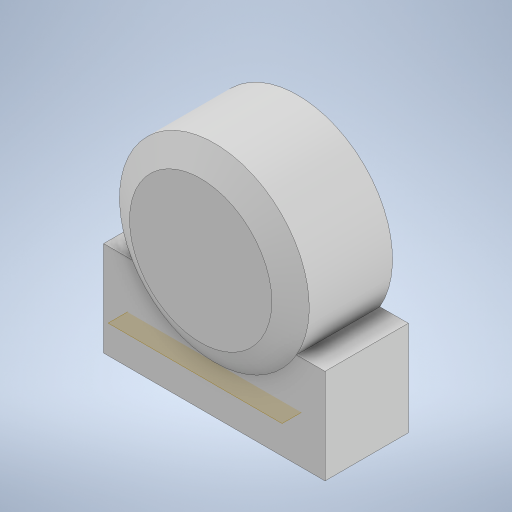
# Autodesk Inventor part: transmission_box_l_to_r
Saved by Autodesk Inventor 2023 (Build 270158000, 158)
## iProperties
Created: 2023-12-09
Part Number: transmission_box_l_to_r
Material: Generic
Document SubType Name: Modeling
Designer: Peter
Density: 1 g/cm^3
Appearance: Default
Author: Peter
Autodesk Inventor part; units mm, degrees
ref_plane "YZ Plane" through (0, 0, 0) normal (1, 0, 0) x (0, 1, 0)
ref_plane "XY Plane" through (0, 0, 0) normal (0, 0, 1) x (1, 0, 0)
sketch "Sketch2" plane through (0, 0, 0) normal (0, 0, 1) x (1, 0, 0)
  circle A0 centre (0, 0) radius 76.2
  dimension "d7" = 152.4
  constraints: 1 centre point, 1 coincident
  measures "d7" diameter of A0
extrude "Extrusion2" add sketch "Sketch2" along normal blind 88.9
chamfer "Chamfer1" distance 19.05 angle 30 1 edges at (-76.2, 0, 88.9) measured on face at (-0.8389, -20.4706, 88.9)
chamfer "Chamfer2" distance 19.05 angle 30 1 edges at (-76.2, 0, 0) measured on face at (-0.8389, -20.4706, 0)
ref_plane "Work Plane1" through (0, -76.2, 0) normal (0, 1, 0) x (-1, 0, 0)
sketch "Sketch10" plane through (0, -76.2, 0) normal (0, 1, 0) x (-1, 0, 0)
  line L0 (88.9, 77.9015) -> (-88.9, 77.9015)
  line L1 (-88.9, 77.9015) -> (-88.9, 10.9985)
  line L2 (-88.9, 10.9985) -> (88.9, 10.9985)
  line L3 (88.9, 10.9985) -> (88.9, 77.9015)
  line L4 (-76.2, 10.9985) -> (76.2, 10.9985) construction
  line L5 (76.2, 77.9015) -> (-76.2, 77.9015) construction
  line L6 (0, -18.1203) -> (0, 108.7218) construction
  dimension "d46" = 88.9
  dimension "d47" = 88.9
  constraints: 8 end point, 2 collinear, 2 parallel, 1 horizontal, 1 perpendicular
  measures "d46" distance between parallel lines of L6 L1
  measures "d47" distance between parallel lines of L3 L6
extrude "Extrusion11" add sketch "Sketch10" along normal mid plane 76.2
body "Solid2"
